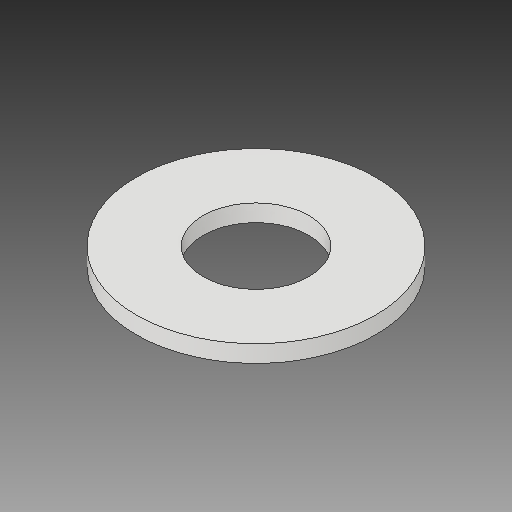
# Autodesk Inventor part: ワッシャー6.2,14.1t
Saved by Autodesk Inventor 2020 (Build 240168000, 168)
## iProperties
Part Number: ワッシャー6.2,14.1t
Material: UHMW、白
Document SubType Name: Modeling
Designer: 雪村
Density: 0.94 g/cm^3
Appearance: 滑らか - 白
Mass: 0.116322 g
Surface Area: 3.10955 cm^2
Volume: 0.123747 cm^3
Author: 雪村
Autodesk Inventor part; units mm, degrees
ref_plane "YZ Plane" through (0, 0, 0) normal (1, 0, 0) x (0, 1, 0)
ref_plane "XZ Plane" through (0, 0, 0) normal (0, 1, 0) x (-1, 0, 0)
ref_plane "XY Plane" through (0, 0, 0) normal (0, 0, 1) x (1, 0, 0)
sketch "スケッチ1" plane through (0, 0, 0) normal (0, 1, 0) x (-1, 0, 0)
  circle A0 centre (0, 0) radius 3.1
  circle A1 centre (0, 0) radius 7
  dimension "d0" = 6.2
  dimension "d1" = 14
  constraints: 2 centre point, 2 coincident
  measures "d0" diameter of A0
  measures "d1" diameter of A1
extrude "押し出し1" add sketch "スケッチ1" along normal blind 1
